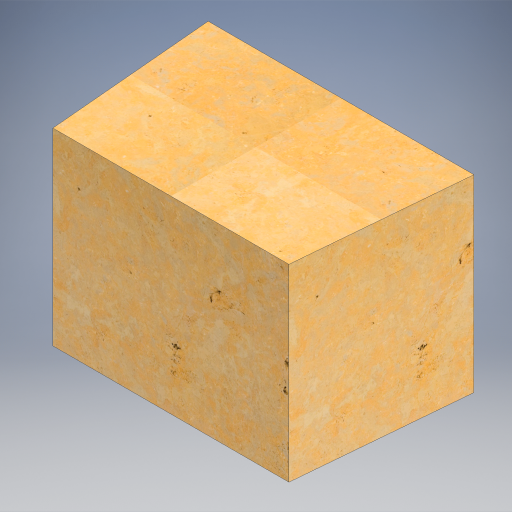
# Autodesk Inventor part: Boulder wall block - 20
Saved by Autodesk Inventor 2023 (Build 270158030, 158C)
## iProperties
RuleStatus: InUse
Created: 2022-05-23
Part Number: Boulder wall block - 20
Material: Granite, Cut, Polished
Document SubType Name: Modeling
Designer: awelt
Mass: 733607 g
Surface Area: 25527.1 cm^2
Volume: 271706 cm^3
Density: 2.7 g/cm^3
Appearance: Amber Select
AfterDocSave0: Convert in3 volume to ft3
in3 to ft3: 0.01
TEST: 0.006
Author: awelt
Autodesk Inventor part; units mm, degrees
ref_plane "YZ Plane" through (0, 0, 0) normal (1, 0, 0) x (0, 1, 0)
ref_plane "XZ Plane" through (0, 0, 0) normal (0, 1, 0) x (-1, 0, 0)
ref_plane "XY Plane" through (0, 0, 0) normal (0, 0, 1) x (1, 0, 0)
sketch "Sketch1" plane through (0, 0, 0) normal (0, 1, 0) x (-1, 0, 0)
  line L0 (-48.0978, -59.8396) -> (-810.7397, -59.8396)
  line L1 (-858.8375, 0) -> (-858.8375, -609.6) construction
  line L2 (-858.8375, -609.6) -> (0, -609.6)
  line L3 (0, -609.6) -> (0, 0) construction
  line L4 (0, -609.6) -> (-48.0978, -59.8396)
  line L5 (-858.8375, -609.6) -> (-810.7397, -59.8396)
  line L6 (-429.4188, -609.6) -> (-429.4187, -59.8396) construction
  dimension "d0" = 858.8375
  dimension "d1" = 609.6
  dimension "d2" = 10
  constraints: 14 end point, 2 midpoint, 2 parallel, 1 horizontal, 1 perpendicular, 1 other
  measures "d0" distance of L2.end L1.end
  measures "d1" distance of L1.end L1.start
  measures "d2" angle of L4 L5
extrude "Extrusion1" add sketch "Sketch1" along normal blind 609.6
body "Solid1"
